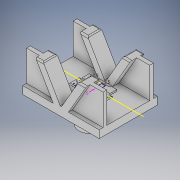
# Autodesk Inventor part: 1.1 Laserhalter Oberteil 20190411.2
Saved by Autodesk Inventor 2018.3 (Build 223284000, 284)
## iProperties
Created: 2018-11-22
Part Number: 1.1 Laserhalter Oberteil 20190411.2
Material: Generisch
Document SubType Name: Modeling
Designer: pgmadmin
Density: 1 g/cm^3
Appearance: Vorgabe
Author: pgmadmin
Autodesk Inventor part; units mm, degrees
ref_plane "YZ Plane" through (0, 0, 0) normal (1, 0, 0) x (0, 1, 0)
ref_plane "XZ Plane" through (0, 0, 0) normal (0, 1, 0) x (-1, 0, 0)
ref_plane "XY Plane" through (0, 0, 0) normal (0, 0, 1) x (1, 0, 0)
sketch "Skizze1" plane through (0, 0, 0) normal (0, 0, 1) x (1, 0, 0)
  line L0 (-25, -19) -> (25, -19)
  line L1 (25, -19) -> (25, 19)
  line L2 (25, 19) -> (-25, 19)
  line L3 (-25, 19) -> (-25, -19)
  line L4 (-25, -19) -> (25, 19) construction
  line L5 (25, -19) -> (-25, 19) construction
  point P0 (0, 0)
  dimension "d0" = 50
  dimension "d1" = 38
  constraints: 12 end point, 2 midpoint, 2 parallel, 1 horizontal, 1 perpendicular
  measures "d0" distance of L1.end L2.end
  measures "d1" distance of L0.end L1.end
extrude "Extrusion1" add sketch "Skizze1" along normal blind 5
sketch "Skizze3" plane through (0, 0, 0) normal (0, 1, 0) x (-1, 0, 0)
  line L0 (25, 5) -> (-25, 5) projected
  line L1 (5, 5) -> (16.547, 25)
  line L2 (-5, 5) -> (-16.547, 25)
  line L3 (16.547, 25) -> (11.547, 25)
  line L4 (-16.547, 25) -> (-11.547, 25)
  line L5 (11.547, 25) -> (0.5, 5.866)
  line L6 (-11.547, 25) -> (-0.5, 5.866)
  line L7 (-0.5, 5.866) -> (0.5, 5.866)
  point P0 (0, 0)
  point P1 (0, 5)
  point P2 (0, 5)
  dimension "d7" = 5
  dimension "d8" = 5
  dimension "d9" = 60
  dimension "d10" = 60
  dimension "d11" = 20
  dimension "d12" = 20
  dimension "d13" = 5
  dimension "d14" = 5
  dimension "d15" = 1
  dimension "d16" = 120
  dimension "d17" = 120
  constraints: 14 end point, 3 horizontal, 2 point on line, 1 coincident, 1 midpoint
  measures "d7" distance of L2.start point (0, 5)
  measures "d8" distance of point (0, 5) L1.start
  measures "d9" angle of L0 L2
  measures "d10" angle of L0 L1
  measures "d11" distance from line of L0 L1.end
  measures "d12" distance from line of L0 L2.end
  measures "d13" distance of L1.end L3.end
  measures "d14" distance of L2.end L4.end
  measures "d15" distance of point (0, 5) L5.end
  measures "d16" angle of L3 L5
  measures "d17" angle of L6 L4
extrude "Extrusion3" add sketch "Skizze3" along normal mid plane 38
sketch "Skizze5" plane through (0, 0, 0) normal (1, 0, 0) x (0, 1, 0)
  line L0 (-19, 5) -> (19, 5) projected
  line L1 (19, 25) -> (-19, 25) projected
  line L2 (10, 5) -> (-10, 5)
  line L3 (-10, 5) -> (-10, 25)
  line L4 (-10, 25) -> (10, 25)
  line L5 (10, 25) -> (10, 5)
  point P0 (0, 0)
  point P1 (19, 5.866)
  dimension "d20" = 20
  dimension "d21" = 9
  constraints: 8 end point, 2 parallel, 2 point on line, 1 horizontal, 1 perpendicular
  measures "d20" distance between parallel lines of L3 L5
  measures "d21" distance from line of point (19, 5.866) L5
extrude "Extrusion4" add sketch "Skizze5" along normal mid plane 50
sketch "Skizze6" plane through (-25, -19, 0) normal (-1, 0, 0) x (0, 0, 1)
  line L0 (25, 29) -> (5, 29) projected
  line L1 (5, 9) -> (5, 0) projected
  line L2 (25, 29) -> (5, 29)
  line L3 (5, 29) -> (5, 9)
  line L4 (5, 9) -> (25, 9)
  line L5 (25, 9) -> (25, 29)
  point P0 (0, 19)
  constraints: 8 end point, 2 parallel, 1 horizontal, 1 perpendicular
extrude "Extrusion5" cut sketch "Skizze6" against normal blind 50
sketch "Skizze7" plane through (0, 0, 5) normal (0, 0, 1) x (1, 0, 0)
  line L0 (0.5, -10) -> (0.5, -19) projected
  line L1 (16.547, -10) -> (16.547, -19) projected
  line L2 (0.5, -16.5) -> (16.547, -16.5)
  line L3 (16.547, -16.5) -> (16.547, -14)
  line L4 (16.547, -14) -> (0.5, -14)
  line L5 (0.5, -14) -> (0.5, -16.5)
  line L6 (16.547, -19) -> (11.547, -19) projected
  line L7 (0.5, 19) -> (0.5, 10) projected
  line L8 (0.5, 14) -> (16.547, 14)
  line L9 (16.547, 14) -> (16.547, 16.5)
  line L10 (16.547, 16.5) -> (0.5, 16.5)
  line L11 (0.5, 16.5) -> (0.5, 14)
  line L12 (11.547, 19) -> (16.547, 19) projected
  line L13 (-0.5, 19) -> (-0.5, 10) projected
  line L14 (-16.547, 19) -> (-16.547, 10) projected
  line L15 (-0.5, 16.5) -> (-16.547, 16.5)
  line L16 (-16.547, 16.5) -> (-16.547, 14)
  line L17 (-16.547, 14) -> (-0.5, 14)
  line L18 (-0.5, 14) -> (-0.5, 16.5)
  line L19 (-11.547, 19) -> (-0.5, 19) projected
  point P0 (0, 0)
  dimension "d30" = 2.5
  dimension "d31" = 2.5
  dimension "d32" = 2.5
  dimension "d33" = 2.5
  dimension "d34" = 2.5
  dimension "d35" = 2.5
  constraints: 24 end point, 6 parallel, 5 point on line, 3 horizontal, 3 perpendicular
  measures "d30" distance between parallel lines of L6 L2
  measures "d31" distance between parallel lines of L4 L2
  measures "d32" distance between parallel lines of L12 L10
  measures "d33" distance between parallel lines of L8 L10
  measures "d34" distance between parallel lines of L15 L19
  measures "d35" distance between parallel lines of L17 L15
sketch "Skizze8" plane through (0, 0, 5) normal (0, 0, 1) x (1, 0, 0)
  line L0 (-0.5, -10) -> (-0.5, -19) projected
  line L1 (-16.547, -10) -> (-16.547, -19) projected
  line L2 (-0.5, -16.5) -> (-16.547, -16.5)
  line L3 (-16.547, -16.5) -> (-16.547, -14)
  line L4 (-16.547, -14) -> (-0.5, -14)
  line L5 (-0.5, -14) -> (-0.5, -16.5)
  line L6 (-25, -19) -> (-5, -19) projected
  point P0 (0, 0)
  dimension "d26" = 2.5
  dimension "d27" = 2.5
  constraints: 8 end point, 2 parallel, 2 point on line, 1 horizontal, 1 perpendicular
  measures "d26" distance between parallel lines of L6 L2
  measures "d27" distance between parallel lines of L2 L4
extrude "Extrusion6" add sketch "Skizze8" along normal blind 20
extrude "Extrusion7" add sketch "Skizze7" along normal blind 20
sketch "Skizze9" plane through (-11.547, -16.5, 25) normal (0, -1, 0) x (1, 0, 0)
  line L0 (11.047, -19.134) -> (11.047, 0) projected
  line L1 (0, 0) -> (11.047, 0) projected
  line L2 (11.047, -19.134) -> (0, 0)
  line L3 (11.047, -19.134) -> (11.047, 0)
  line L4 (0, 0) -> (11.047, 0)
  point P0 (11.547, -25)
  constraints: 6 end point, 1 collinear, 1 vertical
extrude "Extrusion8" cut sketch "Skizze9" against normal blind 50
sketch "Skizze10" plane through (0.5, -16.5, 25) normal (0, -1, 0) x (1, 0, 0)
  line L0 (0, -19.134) -> (0, 0) projected
  line L1 (0, -19.134) -> (0, 0)
  line L2 (0, 0) -> (11.047, 0) projected
  line L3 (0, 0) -> (11.047, 0)
  line L4 (0, -19.134) -> (11.047, 0)
  point P0 (-0.5, -25)
  constraints: 6 end point, 2 collinear
extrude "Extrusion9" cut sketch "Skizze10" against normal blind 50
sketch "Skizze11" plane through (0, 0, 5) normal (0, 0, 1) x (1, 0, 0)
  line L0 (5, -7.5) -> (-5, -7.5)
  line L1 (-5, -7.5) -> (-5, 7.5)
  line L2 (-5, 7.5) -> (5, 7.5)
  line L3 (5, 7.5) -> (5, -7.5)
  line L4 (5, -7.5) -> (-5, 7.5) construction
  line L5 (-5, -7.5) -> (5, 7.5) construction
  point P0 (0, 0)
  dimension "d42" = 15
  dimension "d43" = 10
  constraints: 12 end point, 2 midpoint, 2 parallel, 1 horizontal, 1 perpendicular
  measures "d42" distance of L0.end L1.end
  measures "d43" distance of L1.end L2.end
extrude "Extrusion10" add sketch "Skizze11" along normal blind 3
sketch "Skizze12" plane through (5, -7.5, 5) normal (1, 0, 0) x (0, 0, -1)
  line L0 (0, 0) -> (0, 15) projected
  line L1 (0, 2.5) -> (-2, 2.5)
  line L2 (-2, 2.5) -> (-2, 12.5)
  line L3 (-2, 12.5) -> (0, 12.5)
  line L4 (0, 12.5) -> (0, 2.5)
  line L5 (0, 15) -> (-3, 15) projected
  point P0 (5, 7.5)
  dimension "d46" = 10
  dimension "d47" = 2.5
  dimension "d48" = 2
  constraints: 8 end point, 2 parallel, 1 horizontal, 1 perpendicular, 1 point on line
  measures "d46" distance of L1.end L2.end
  measures "d47" distance between parallel lines of L5 L3
  measures "d48" distance between parallel lines of L0 L2
extrude "Extrusion11" cut sketch "Skizze12" against normal blind 15
sketch "Skizze13" plane through (0, 0, 8) normal (0, 0, 1) x (1, 0, 0)
  line L0 (-5, 5) -> (-5, -5) projected
  line L1 (5, -5) -> (5, 5) projected
  line L2 (-35, 0) -> (35, 0) projected
  line L3 (5, 5) -> (-5, 5) projected
  line L4 (-5, -5) -> (-2.5, -5)
  line L5 (-2.5, -5) -> (-2.5, 5)
  line L6 (-2.5, 5) -> (-5, 5)
  line L7 (-5, 5) -> (-5, -5)
  line L8 (5, -5) -> (5, -7.5) projected
  line L9 (5, -5) -> (2.5, -5)
  line L10 (2.5, -5) -> (2.5, 5)
  line L11 (2.5, 5) -> (5, 5)
  line L12 (5, 5) -> (5, -5)
  point P0 (0, 0)
  point P1 (-5, -5)
  dimension "d51" = 5
  dimension "d52" = 5
  dimension "d53" = 2.5
  dimension "d54" = 2.5
  constraints: 16 end point, 4 parallel, 4 point on line, 2 horizontal, 2 perpendicular
  measures "d51" distance from line of L2 point (-5, -5)
  measures "d52" distance from line of L2 L8.start
  measures "d53" distance of L6.end L5.end
  measures "d54" distance of L10.end L11.end
fillet "Rundung3" radius 1 12 edges at (14.047, -19, 25) (11.547, -14.5, 25) (14.047, -10, 25) (-14.047, -19, 25) (-11.547, -14.5, 25) (-14.047, -10, 25) (-14.047, 10, 25) (-11.547, 14.5, 25) (-14.047, 19, 25) (11.547, 14.5, 25) (14.047, 19, 25) (14.047, 10, 25)
sketch "Skizze14" plane through (0, 0, 5) normal (0, 0, 1) x (1, 0, 0)
  line L0 (16.547, -14) -> (16.547, -16.5) projected
  line L1 (25, -19) -> (25, 19) projected
  line L2 (16.547, -16.5) -> (25, -16.5)
  line L3 (25, -16.5) -> (25, -14)
  line L4 (25, -14) -> (16.547, -14)
  line L5 (16.547, -14) -> (16.547, -16.5)
  line L6 (-16.547, -16.5) -> (-16.547, -18) projected
  line L7 (-25, 19) -> (-25, -19) projected
  line L8 (-16.547, -16.5) -> (-25, -16.5)
  line L9 (-25, -16.5) -> (-25, -14)
  line L10 (-25, -14) -> (-16.547, -14)
  line L11 (-16.547, -14) -> (-16.547, -16.5)
  line L12 (-16.547, 16.5) -> (-16.547, 14) projected
  line L13 (-16.547, 16.5) -> (-25, 16.5)
  line L14 (-25, 16.5) -> (-25, 14)
  line L15 (-25, 14) -> (-16.547, 14)
  line L16 (-16.547, 14) -> (-16.547, 16.5)
  line L17 (16.547, 16.5) -> (16.547, 14) projected
  line L18 (16.547, 16.5) -> (25, 16.5)
  line L19 (25, 16.5) -> (25, 14)
  line L20 (25, 14) -> (16.547, 14)
  line L21 (16.547, 14) -> (16.547, 16.5)
  point P0 (0, 0)
  dimension "d63" = 2.5
  dimension "d64" = 2.5
  dimension "d65" = 2.5
  dimension "d66" = 2.5
  constraints: 32 end point, 8 parallel, 4 horizontal, 4 perpendicular, 4 point on line
  measures "d63" distance between parallel lines of L2 L4
  measures "d64" distance between parallel lines of L8 L10
  measures "d65" distance between parallel lines of L13 L15
  measures "d66" distance between parallel lines of L18 L20
extrude "Extrusion13" add sketch "Skizze14" along normal blind 20
sketch "Skizze17" plane through (0, 0, 5) normal (0, 0, 1) x (1, 0, 0)
  line L0 (-5, 8.5) -> (-9, 8.5)
  line L1 (-9, 8.5) -> (-9, 4)
  line L2 (-9, 4) -> (-5, 4)
  line L3 (-5, 4) -> (-5, 8.5)
  line L4 (5, 7.5) -> (-5, 7.5) projected
  line L5 (-5, 5) -> (-2.366, 5) projected
  line L6 (-5, 7.5) -> (-5, -7.5) projected
  line L7 (5, 8.5) -> (9, 8.5)
  line L8 (9, 8.5) -> (9, 4)
  line L9 (9, 4) -> (5, 4)
  line L10 (5, 4) -> (5, 8.5)
  line L11 (-5, -4) -> (-9, -4)
  line L12 (-9, -4) -> (-9, -8.5)
  line L13 (-9, -8.5) -> (-5, -8.5)
  line L14 (-5, -8.5) -> (-5, -4)
  line L15 (-2.366, -5) -> (-5, -5) projected
  line L16 (5, -4) -> (9, -4)
  line L17 (9, -4) -> (9, -8.5)
  line L18 (9, -8.5) -> (5, -8.5)
  line L19 (5, -8.5) -> (5, -4)
  line L20 (5, -5) -> (2.366, -5) projected
  line L21 (25, -14) -> (25, 14) projected
  point P0 (0, 0)
  point P1 (0, -7.5577)
  dimension "d88" = 1
  dimension "d89" = 1
  dimension "d90" = 4
  dimension "d91" = 0
  dimension "d92" = 4
  dimension "d93" = 4.5
  dimension "d94" = 10
  dimension "d95" = 1
  dimension "d96" = 4
  dimension "d97" = 4.5
  dimension "d98" = 1
  dimension "d99" = 4
  dimension "d100" = 4.5
  dimension "d101" = 10
  dimension "d102" = 5
  dimension "d103" = 1
  dimension "d104" = 25
  constraints: 32 end point, 8 parallel, 4 horizontal, 4 perpendicular
  measures "d88" distance between parallel lines of L4 L0
  measures "d89" distance between parallel lines of L5 L2
  measures "d90" distance between parallel lines of L3 L1
  measures "d91" distance between parallel lines of L6 L3
  measures "d92" distance between parallel lines of L8 L10
  measures "d93" distance between parallel lines of L9 L7
  measures "d94" distance between parallel lines of L3 L10
  measures "d95" distance between parallel lines of L4 L7
  measures "d96" distance of L11.start L11.end
  measures "d97" distance between parallel lines of L13 L11
  measures "d98" distance between parallel lines of L15 L11
  measures "d99" distance of L16.start L16.end
  measures "d100" distance of L16.end L17.end
  measures "d101" distance between parallel lines of L19 L14
  measures "d102" distance from line of L14 point (0, -7.558)
  measures "d103" distance between parallel lines of L20 L16
  measures "d104" distance from line of L21 point (0, -7.558)
extrude "Extrusion15" add sketch "Skizze17" along normal blind 2 contours L3 L2 L1 L0 | L7 L8 L9 L10 | L16 L17 L18 L19
sketch "Skizze18" plane through (0, 0, 0) normal (0, 0, -1) x (-1, 0, 0)
  circle A0 centre (0, 0) radius 7.25
  dimension "d110" = 14.5
  constraints: 1 centre point, 1 coincident
  measures "d110" diameter of A0
extrude "Extrusion16" add sketch "Skizze18" along normal blind 14
sketch "Skizze20" plane through (0, 0, 8) normal (0, 0, 1) x (1, 0, 0)
  line L0 (-5, -7.5) -> (5, -7.5) projected
  line L1 (5, 8.5) -> (5, 7.5) projected
  line L2 (-5, -7.5) -> (5, -7.5)
  line L3 (5, -7.5) -> (5, 7.4941)
  line L4 (5, 7.4941) -> (-5, 7.4941)
  line L5 (-5, 7.4941) -> (-5, -7.5)
  point P0 (0, 0)
  point P1 (5, 4)
  constraints: 8 end point, 2 parallel, 1 horizontal, 1 perpendicular, 1 point on line
extrude "Extrusion18" add sketch "Skizze20" along normal blind 1
sketch "Skizze21" plane through (0, 0, 5) normal (0, 0, 1) x (1, 0, 0)
  line L0 (-9, 4) -> (-5, 4) projected
  line L1 (9, -4) -> (-9, -4)
  line L2 (-9, -4) -> (-9, 4)
  line L3 (-9, 4) -> (9, 4)
  line L4 (9, 4) -> (9, -4)
  line L5 (9, -4) -> (-9, 4) construction
  line L6 (-9, -4) -> (9, 4) construction
  point P0 (0, 0)
  constraints: 12 end point, 2 midpoint, 2 parallel, 1 horizontal, 1 perpendicular
extrude "Extrusion19" cut sketch "Skizze21" against normal blind 2
sketch "Skizze22" plane through (0, 0, 5) normal (0, 0, 1) x (1, 0, 0)
  line L0 (5, -4) -> (-9, -4) projected
  line L1 (-9, -4) -> (-5, -4)
  line L2 (-5, -4) -> (-5, -8.5)
  line L3 (-5, -8.5) -> (-9, -8.5)
  line L4 (-9, -8.5) -> (-9, -4)
  point P0 (0, 0)
  dimension "d119" = 4.5
  dimension "d120" = 4
  constraints: 8 end point, 2 parallel, 1 horizontal, 1 perpendicular
  measures "d119" distance of L3.end L0.end
  measures "d120" distance of L2.end L3.end
extrude "Extrusion20" add sketch "Skizze22" along normal blind 2
sketch "Skizze23" plane through (-5, 5, 7) normal (-1, 0, 0) x (0, 0, 1)
  line L0 (2, 2.4941) -> (2, -12.5) projected
  line L1 (2, 2.4941) -> (1, 2.4941)
  line L2 (1, 2.4941) -> (1, -12.5)
  line L3 (1, -12.5) -> (2, -12.5)
  line L4 (2, -12.5) -> (2, 2.4941)
  point P0 (-7, -5)
  dimension "d123" = 1
  constraints: 8 end point, 2 parallel, 1 horizontal, 1 perpendicular
  measures "d123" distance between parallel lines of L0 L2
extrude "Extrusion21" cut sketch "Skizze23" against normal blind 10
sketch "Skizze24" plane through (-9, 4, 7) normal (-1, 0, 0) x (0, 0, 1)
  line L0 (-2, 4.5) -> (0, 4.5) projected
  line L1 (-1, 4.5) -> (1, 4.5)
  line L2 (1, 4.5) -> (1, -12.5)
  line L3 (1, -12.5) -> (-1, -12.5)
  line L4 (-1, -12.5) -> (-1, 4.5)
  line L5 (1, 3.5) -> (1, -11.5) projected
  point P0 (-7, -4)
  dimension "d126" = 2
  dimension "d127" = 0
  dimension "d128" = 17
  constraints: 8 end point, 2 parallel, 1 horizontal, 1 midpoint, 1 perpendicular
  measures "d126" distance of L2.end L3.end
  measures "d127" distance between parallel lines of L5 L2
  measures "d128" distance of L3.end L1.start
extrude "Extrusion22" cut sketch "Skizze24" against normal blind 20
fillet "Rundung4" radius 2 1 edges at (-9, 0, 5)
fillet "Rundung5" radius 2 1 edges at (9, 0, 5)
sketch "Skizze25" plane through (-5, 4, 5) normal (0, -1, 0) x (1, 0, 0)
  point P0 (5, -5)
sketch "Skizze26" plane through (-5, 5, 5) normal (0, -1, 0) x (1, 0, 0)
  line L0 (10, 0) -> (0, 0) projected
  line L1 (10, 1) -> (0, 1) projected
  line L2 (10, 0) -> (0, 0)
  line L3 (0, 0) -> (0, 1)
  line L4 (0, 1) -> (10, 1)
  line L5 (10, 1) -> (10, 0)
  point P0 (5, -5)
  constraints: 8 end point, 2 parallel, 1 horizontal, 1 perpendicular
extrude "Extrusion23" add sketch "Skizze26" along normal blind 11
sketch "Skizze27" plane through (9, -4, 6) normal (0, 1, 0) x (1, 0, 0)
  line L0 (7.547, -19) -> (-4, 1) projected
  line L1 (-4, 1) -> (-15, 1)
  line L2 (-15, 1) -> (-15, 2)
  line L3 (-15, 2) -> (-4, 2)
  line L4 (-4, 2) -> (-4, 1)
  point P0 (-9, 6)
  dimension "d135" = 11
  dimension "d136" = 1
  constraints: 8 end point, 2 parallel, 1 horizontal, 1 perpendicular
  measures "d135" distance of L2.end L3.end
  measures "d136" distance of L1.end L2.end
extrude "Extrusion24" add sketch "Skizze27" along normal blind 11
sketch "Skizze28" plane through (-6, -4, 5) normal (0, 0, 1) x (1, 0, 0)
  line L0 (0, 8) -> (1, 8) projected
  line L1 (0, 0) -> (0, 8) projected
  line L2 (1, 8) -> (0, 8)
  line L3 (0, 8) -> (0, 0)
  line L4 (0, 0) -> (1, 0)
  line L5 (1, 0) -> (1, 8)
  point P0 (6, 4)
  constraints: 8 end point, 2 parallel, 1 horizontal, 1 perpendicular
extrude "Extrusion25" cut sketch "Skizze28" against normal blind 1
